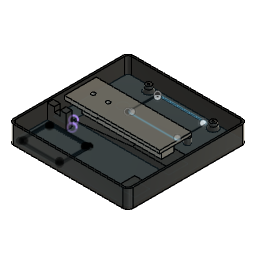
ESPressoScale_Mavin_NA27 (Autodesk Fusion 360 design; units mm, degrees)
Autodesk Fusion 360 part; units mm, degrees
note: some values were not read from the file. Set by a fixed rule: which face or edge a step refers to.
sketch "Skizze1" plane through (0, 0, 0) normal (0, 0, 1) x (1, 0, 0)
  line L0 (-40, 6.35) -> (40, 6.35)
  line L1 (40, 6.35) -> (40, -6.35)
  line L2 (40, -6.35) -> (-40, -6.35)
  line L3 (-40, -6.35) -> (-40, 6.35)
  circle A0 centre (-35, 0.002) radius 2
  circle A1 centre (-20, 0.002) radius 2
  circle A2 centre (35, 0.002) radius 2.5
  circle A3 centre (20, 0.002) radius 2.5
  dimension "d1" = 80
  dimension "d2" = 12.7
  dimension "d3" = 6.35
  dimension "d4" = 40
  dimension "d5" = 4
  dimension "d6" = 5
  dimension "d7" = 4
  dimension "d8" = 20
  dimension "d9" = 5
  dimension "d10" = 5
  dimension "d11" = 5
  dimension "d12" = 20
  constraint horizontal L0
  constraint vertical L1
  constraint horizontal L2
  constraint vertical L3
  measures "d1" distance of L0.start L0.end
  measures "d2" distance of L0.start L2.end
  measures "d3" distance of origin L0
  measures "d4" distance of origin L1
  measures "d5" diameter of A0
  measures "d6" distance of L3 A0.centre
  measures "d7" diameter of A1
  measures "d8" distance of L3 A1.centre
  measures "d9" diameter of A2
  measures "d10" distance of L1 A2.centre
  measures "d11" diameter of A3
  measures "d12" distance of L1 A3.centre
extrude "Extrusion1" add sketch "Skizze1" along normal blind 12.7 makes body 1
copy_body "Körper->Berechn1" bodies 1 removing the originals makes body 2 in component "300gWaegezelle"
sketch "Skizze2" plane through (0, 0, 0) normal (0, 0, 1) x (1, 0, 0)
  line L0 (-65, 65) -> (65, 65)
  line L1 (65, 65) -> (65, -65)
  line L2 (65, -65) -> (-65, -65)
  line L3 (-65, -65) -> (-65, 65)
  dimension "d15" = 130
  dimension "d16" = 130
  dimension "d17" = 65
  dimension "d18" = 65
  constraint horizontal L0
  constraint vertical L1
  constraint horizontal L2
  constraint vertical L3
  measures "d15" distance of L0.start L0.end
  measures "d16" distance of L0.start L2.end
  measures "d17" distance of origin L0
  measures "d18" distance of origin L3
ref_plane "Arbeitsebene1" through (0, 0, 25) normal (0, 0, 1) x (1, 0, 0)
extrude "Extrusion2" add sketch "Skizze2" against normal blind 20 from surface at 25 separate body makes body 3
fillet "Abrundung1" radius 5 8 edges at (-65, 0, 25) (0, 65, 25) (65, 0, 25) (0, -65, 25) (65, -65, 15) (-65, -65, 15) (-65, 65, 15) (65, 65, 15) on bodies 3
shell "Schale1" thickness 3 removed faces 1 at (-23.3333, -21.6667, 5) on bodies 3
extrude "Extrusion3" add 1 faces at (-20, 20, 22) along direction (0, 0, 1) blind 18 from surface at -22 on bodies 3 bodies 3 makes body 4
fillet "Abrundung2" radius 5 4 edges at (60, 60, 9) (-60, 60, 9) (-60, -60, 9) (60, -60, 9) on bodies 4
shell "Schale2" thickness 1.6 outward thickness 0.2 removed faces 1 at (18.3333, -20, 18) on bodies 4
move_body "Verschieben1" bodies 2 to x (1, 0, 0) y (0, 1, 0) z (0, 0, 1) at (0, 0, 8) in component "300gWaegezelle"
sketch "Skizze3" plane through (0, 0, 25) normal (0, 0, 1) x (-1, 0, 0)
  line L0 (60, 60) -> (-60, 60)
  line L1 (-60, 60) -> (-60, -60)
  line L2 (-60, -60) -> (60, -60)
  line L3 (60, -60) -> (60, 60)
  circle A0 centre (0, 0) radius 22
  line L4 (45, 35) -> (31, 35)
  line L5 (31, 35) -> (31, 53)
  line L6 (31, 53) -> (45, 53)
  line L7 (45, 53) -> (45, 35)
  line L8 (-45, 35) -> (-31, 35)
  line L9 (-31, 35) -> (-31, 53)
  line L10 (-31, 53) -> (-45, 53)
  line L11 (-45, 53) -> (-45, 35)
  line L12 (12, 38) -> (-12, 38)
  line L13 (-12, 38) -> (-12, 53)
  line L14 (-12, 53) -> (12, 53)
  line L15 (12, 53) -> (12, 38)
  line L16 (12, 53) -> (-15, 53)
  line L17 (20, 33) -> (-20, 33)
  line L18 (-20, 33) -> (-20, 29)
  line L19 (-20, 29) -> (20, 29)
  line L20 (20, 29) -> (20, 33)
  dimension "d33" = 44
  dimension "d39" = 14
  dimension "d40" = 18
  dimension "d41" = 15
  dimension "d42" = 95
  dimension "d43" = 14
  dimension "d44" = 18
  dimension "d45" = 95
  dimension "d46" = 15
  dimension "d47" = 24
  dimension "d48" = 15
  dimension "d49" = 12
  dimension "d50" = 98
  dimension "d93" = 7
  dimension "d94" = 7
  dimension "d111" = 40
  dimension "d112" = 4
  dimension "d113" = 20
  dimension "d114" = 20
  constraint coincident A0.centre origin
  constraint horizontal L4
  constraint vertical L5
  constraint horizontal L6
  constraint vertical L7
  constraint horizontal L8
  constraint vertical L9
  constraint horizontal L10
  constraint vertical L11
  constraint horizontal L12
  constraint vertical L13
  constraint horizontal L14
  constraint vertical L15
  constraint horizontal L16
  constraint horizontal L17
  constraint vertical L18
  constraint horizontal L19
  constraint vertical L20
  measures "d33" diameter of A0
  measures "d39" distance of L4.start L4.end
  measures "d40" distance of L4.start L6.end
  measures "d41" distance of L3 L7
  measures "d42" distance of L2 L4
  measures "d43" distance of L8.start L8.end
  measures "d44" distance of L8.start L10.end
  measures "d45" distance of L2 L8
  measures "d46" distance of L1 L11
  measures "d47" distance of L12.start L12.end
  measures "d48" distance of L12.start L14.end
  measures "d49" distance of A0.centre L15
  measures "d50" distance of L2 L12
  measures "d93" distance of L0 L14
  measures "d94" distance of L0 L6
  measures "d111" distance of L17.start L17.end
  measures "d112" distance of L17.start L19.end
  measures "d113" distance of A0.centre L18
  measures "d114" distance of L16 L17
extrude "Extrusion5" cut sketch "Skizze3" against normal blind 1 contours A0 bodies 3
extrude "Extrusion6" cut sketch "Skizze3" against normal blind 10 contours L12 L13 L14 L15 L16 bodies 3
extrude "Extrusion7" cut sketch "Skizze3" along normal blind 1.8 from surface at -3 contours L4 L5 L6 L7 | L8 L9 L10 L11 bodies 3
sketch "Skizze4" plane through (0, 0, 1.6) normal (0, 0, 1) x (-1, 0, 0)
  arc A0 (-55, 58.4) -> (-58.4, 55) centre (-55, 55) ccw
  line L0 (-58.4, 55) -> (-58.4, -55)
  arc A1 (-58.4, -55) -> (-55, -58.4) centre (-55, -55) ccw
  line L1 (-55, -58.4) -> (55, -58.4)
  arc A2 (55, -58.4) -> (58.4, -55) centre (55, -55) ccw
  line L2 (58.4, -55) -> (58.4, 55)
  arc A3 (58.4, 55) -> (55, 58.4) centre (55, 55) ccw
  line L3 (55, 58.4) -> (-55, 58.4)
  line L4 (-48.8958, 7.8489) -> (-13.942, 7.8489)
  line L5 (-13.942, 7.8489) -> (-13.942, -7.6745)
  line L6 (-13.942, -7.6745) -> (-48.8958, -7.6745)
  line L7 (-48.8958, -7.6745) -> (-48.8958, 7.8489)
  circle A4 centre (-34.9997, -0.0031) radius 2.75
  circle A5 centre (-19.9963, -0.0044) radius 2.75
  circle A6 centre (-32.5, -53.4) radius 1
  circle A7 centre (-32.5, -53.4) radius 3
  circle A8 centre (32.5, -53.4) radius 1
  circle A9 centre (32.5, -53.4) radius 3
  circle A10 centre (-32.5, -27.4) radius 1
  circle A11 centre (-32.5, -27.4) radius 3
  circle A12 centre (32.5, -27.4) radius 1
  circle A13 centre (32.5, -27.4) radius 3
  line L8 (-53.4, 46.6) -> (-38.4, 46.6)
  line L9 (-38.4, 46.6) -> (-38.4, 31.6)
  line L10 (-38.4, 31.6) -> (-53.4, 31.6)
  line L11 (-53.4, 31.6) -> (-53.4, 46.6)
  line L12 (-55.4, 48.6) -> (-36.4, 48.6)
  line L13 (-36.4, 48.6) -> (-36.4, 29.6)
  line L14 (-36.4, 29.6) -> (-55.4, 29.6)
  line L15 (-55.4, 29.6) -> (-55.4, 48.6)
  line L16 (57.4, 23) -> (37.4, 23)
  line L17 (37.4, 23) -> (37.4, 17)
  line L18 (37.4, 17) -> (57.4, 17)
  line L19 (57.4, 17) -> (57.4, 23)
  line L20 (51.4, 23) -> (45.4, 23)
  line L21 (45.4, 23) -> (45.4, 17)
  line L22 (45.4, 17) -> (51.4, 17)
  line L23 (51.4, 17) -> (51.4, 23)
  circle A14 centre (-34.9997, -0.0031) radius 5.25
  circle A15 centre (-19.9963, -0.0044) radius 5.25
  dimension "d56" = 5.5
  dimension "d57" = 5.5
  dimension "d58" = 2
  dimension "d59" = 32.5
  dimension "d60" = 6
  dimension "d63" = 65
  dimension "d64" = 26
  dimension "d72" = 15
  dimension "d73" = 15
  dimension "d74" = 5
  dimension "d75" = 90
  dimension "d76" = 96.8
  dimension "d77" = -2
  dimension "d80" = 5
  dimension "d81" = 20
  dimension "d82" = 6
  dimension "d83" = 23
  dimension "d84" = 1
  dimension "d85" = 6
  dimension "d86" = 6
  dimension "d118" = 10.5
  dimension "d119" = 10.5
  constraint horizontal L4
  constraint vertical L5
  constraint horizontal L6
  constraint vertical L7
  constraint concentric A6 A7
  constraint horizontal L8
  constraint vertical L9
  constraint horizontal L10
  constraint vertical L11
  constraint horizontal L16
  constraint vertical L17
  constraint horizontal L18
  constraint vertical L19
  constraint horizontal L20
  constraint vertical L21
  constraint horizontal L22
  constraint vertical L23
  constraint coincident L16 L20.start
  constraint concentric A4 A14
  constraint concentric A5 A15
  measures "d56" diameter of A4
  measures "d57" diameter of A5
  measures "d58" diameter of A6
  measures "d59" horizontal distance of origin A6.centre
  measures "d60" diameter of A7
  measures "d72" distance of L8.start L8.end
  measures "d73" distance of L8.start L10.end
  measures "d74" distance of L0 L11
  measures "d75" distance of L1 L10
  measures "d76" distance of L2 L9
  measures "d80" distance of L1 A6.centre
  measures "d81" distance of L16.start L16.end
  measures "d82" distance of L16.start L18.end
  measures "d83" distance of origin L16
  measures "d84" distance of L2 L19
  measures "d85" distance of L20.start L20.end
  measures "d86" distance of L19 L23
  measures "d118" diameter of A14
  measures "d119" diameter of A15
extrude "Extrusion1'" add sketch "Skizze4" along normal up to surface (6.4 mm away) separate body contours L4 L5 L6 L7 | A14 | A15 makes body 5 in component "300gWaegezelle"
combine "Kombinieren1" operation add target body 4 tool bodies 5
move_face "Flächen versetzen1" offset 2 1 faces at (25.5932, 7.6745, 3.7333) on bodies 4
move_face "Flächen versetzen2" offset 2 1 faces at (48.8958, 3.8333, 3.7333) on bodies 4
move_face "Flächen versetzen3" offset 2 1 faces at (38.5779, -7.8489, 3.7333) on bodies 4
extrude "Extrusion8" add sketch "Skizze4" along normal blind 6 contours A7 | A9 | A11 | A13 bodies 4
extrude "Extrusion9" add sketch "Skizze4" along normal blind 4 contours L8 L9 L10 L11 bodies 4
extrude "Extrusion10" add sketch "Skizze4" along normal blind 15 contours L16 L18 L19 L23 | L16 L17 L18 L21 bodies 4
extrude "Extrusion11" add sketch "Skizze4" along normal blind 10 contours L16 L18 L20 L21 L22 L23 bodies 4
sketch "Skizze5" plane through (0, 0, 22) normal (0, 0, -1) x (1, 0, 0)
  line L0 (60, 60) -> (-60, 60)
  line L1 (-60, 60) -> (-60, -60)
  line L2 (-60, -60) -> (60, -60)
  line L3 (60, -60) -> (60, 60)
  line L4 (12, 53) -> (12, 38)
  line L5 (12, 38) -> (-12, 38)
  line L6 (-12, 38) -> (-12, 53)
  line L7 (-45, 53) -> (-31, 53)
  line L8 (-31, 53) -> (-31, 35)
  line L9 (-31, 35) -> (-45, 35)
  line L10 (-45, 35) -> (-45, 53)
  line L11 (45, 53) -> (45, 35)
  line L12 (45, 35) -> (31, 35)
  line L13 (31, 35) -> (31, 53)
  line L14 (31, 53) -> (45, 53)
  line L15 (-17.5, 55) -> (17.5, 55)
  line L16 (17.5, 55) -> (17.5, 35)
  line L17 (17.5, 35) -> (-17.5, 35)
  line L18 (-17.5, 35) -> (-17.5, 55)
  line L19 (-12, 53) -> (12, 53)
  line L20 (-17.5, 55) -> (17.5, 55)
  line L21 (17.5, 55) -> (17.5, 63)
  line L22 (17.5, 63) -> (-17.5, 63)
  line L23 (-17.5, 63) -> (-17.5, 55)
  dimension "d102" = 35
  dimension "d103" = 20
  dimension "d104" = 17.5
  dimension "d105" = 5
  dimension "d125" = 8
  constraint horizontal L15
  constraint vertical L16
  constraint horizontal L17
  constraint vertical L18
  constraint horizontal L20
  constraint vertical L21
  constraint horizontal L22
  constraint vertical L23
  measures "d102" distance of L15.start L15.end
  measures "d103" distance of L15.start L17.end
  measures "d104" distance of origin L16
  measures "d105" distance of L0 L15
  measures "d125" distance of L15.start L22.end
extrude "Extrusion13" cut sketch "Skizze5" against normal blind 1.5 contours L15 L16 L17 L18 L20 bodies 3
extrude "Extrusion14" add sketch "Skizze3" against normal blind 1.5 from surface at -3 contours L17 L18 L19 L20 bodies 3
chamfer "Fase1" distance 59 distance2 6.4 1 edges at (13.942, -0.0872, 1.6) measured on face at (-18, -42.6667, 1.6) on bodies 4
extrude "Extrusion15" cut sketch "Skizze4" along normal blind 5 from surface at -1.8 contours A4 | A5 | A14 | A15 bodies 4
extrude "Extrusion16" add sketch "Skizze5" along normal blind 1.5 contours L0 L15 L20 L21 L23 | L0 L21 L22 L23 bodies 3
extrude "Extrusion17" add sketch "Skizze5" against normal blind 0.7 separate body contours L15 L16 L17 L18 L20 makes body 6
extrude "Extrusion18" add sketch "Skizze5" against normal blind 2 contours L4 L5 L6 L19 bodies 6
extrude "Extrusion19" cut 1 faces at (-37.4, -21, 11.6) along direction (-1, 0, 0) blind 2 on bodies 4 bodies 4
chamfer "Fase3" distance 2 distance2 3 3 edges at (-29.703, 52.3152, 1.6) (-29.703, 26.3152, 1.6) (35.297, 52.3152, 1.6) measured on face at (-18.6667, -42.6667, 1.6) measured on face at (-18.6667, -42.6667, 1.6) measured on face at (-18.6667, -42.6667, 1.6) on bodies 4
extrude "Extrusion20" add 1 faces at (-57.4, -19, 11.6) along direction (-1, 0, 0) up to surface (1 mm away) on bodies 4 bodies 4
sketch "Skizze7" plane through (0, 0, 1.6) normal (0, 0, 1) x (-1, 0, 0)
  line L0 (45.058, -9.6745) -> (-50.8958, -9.6745)
  line L1 (-50.8958, -9.6745) -> (-50.8958, 9.8489)
  line L2 (-50.8958, 9.8489) -> (45.058, 9.8489)
  line L3 (45.058, 9.8489) -> (45.058, -9.6745)
  line L4 (-53.4, 31.6) -> (-53.4, 46.6)
  line L5 (-53.4, 46.6) -> (-38.4, 46.6)
  line L6 (-38.4, 46.6) -> (-38.4, 31.6)
  line L7 (-38.4, 31.6) -> (-53.4, 31.6)
  line L8 (39.4, 23) -> (58.4, 23)
  line L9 (58.4, 23) -> (58.4, 55)
  arc A0 (58.4, 55) -> (55, 58.4) centre (55, 55) ccw
  line L10 (55, 58.4) -> (-55, 58.4)
  arc A1 (-55, 58.4) -> (-58.4, 55) centre (-55, 55) ccw
  line L11 (-58.4, 55) -> (-58.4, -55)
  arc A2 (-58.4, -55) -> (-55, -58.4) centre (-55, -55) ccw
  line L12 (-55, -58.4) -> (-32.5, -58.4)
  circle A3 centre (-32.5, -53.4) radius 5
  line L13 (-32.5, -58.4) -> (32.5, -58.4)
  circle A4 centre (32.5, -53.4) radius 5
  line L14 (32.5, -58.4) -> (55, -58.4)
  arc A5 (55, -58.4) -> (58.4, -55) centre (55, -55) ccw
  line L15 (58.4, -55) -> (58.4, 17)
  line L16 (58.4, 17) -> (39.4, 17)
  line L17 (39.4, 17) -> (39.4, 23)
  circle A6 centre (-32.5, -27.4) radius 3
  circle A7 centre (32.5, -27.4) radius 5
  line L18 (23, -54.7754) -> (-23, -54.7754)
  line L19 (-25, -52.7754) -> (-25, -26.7754)
  line L20 (-23, -24.7754) -> (23, -24.7754)
  line L21 (25, -26.7754) -> (25, -52.7754)
  line L22 (16, 55) -> (52, 55)
  line L23 (54, 53) -> (54, 27)
  line L24 (52, 25) -> (16, 25)
  line L25 (14, 27) -> (14, 53)
  arc A8 (52, 25) -> (54, 27) centre (52, 27) ccw
  arc A9 (14, 27) -> (16, 25) centre (16, 27) ccw
  arc A10 (16, 55) -> (14, 53) centre (16, 53) ccw
  arc A11 (54, 53) -> (52, 55) centre (52, 53) ccw
  line L26 (52, 26) -> (16, 26)
  arc A12 (15, 27) -> (16, 26) centre (16, 27) ccw
  line L27 (15, 27) -> (15, 53)
  arc A13 (16, 54) -> (15, 53) centre (16, 53) ccw
  line L28 (16, 54) -> (52, 54)
  arc A14 (53, 53) -> (52, 54) centre (52, 53) ccw
  line L29 (53, 53) -> (53, 27)
  arc A15 (52, 26) -> (53, 27) centre (52, 27) ccw
  arc A16 (12.5, 27) -> (16, 23.5) centre (16, 27) ccw
  line L30 (52, 23.5) -> (16, 23.5)
  arc A17 (52, 23.5) -> (55.5, 27) centre (52, 27) ccw
  line L31 (55.5, 53) -> (55.5, 27)
  arc A18 (55.5, 53) -> (52, 56.5) centre (52, 53) ccw
  line L32 (16, 56.5) -> (52, 56.5)
  arc A19 (16, 56.5) -> (12.5, 53) centre (16, 53) ccw
  line L33 (12.5, 27) -> (12.5, 53)
  arc A20 (23, -54.7754) -> (25, -52.7754) centre (23, -52.7754) ccw
  arc A21 (-25, -52.7754) -> (-23, -54.7754) centre (-23, -52.7754) ccw
  arc A22 (-23, -24.7754) -> (-25, -26.7754) centre (-23, -26.7754) ccw
  arc A23 (25, -26.7754) -> (23, -24.7754) centre (23, -26.7754) ccw
  point P0 (25, -54.7754)
  point P1 (25, -24.7754)
  point P2 (14, 55)
  point P3 (54, 55)
  point P4 (14, 25)
  dimension "d140" = 30
  dimension "d141" = 50
  dimension "d142" = 25
  dimension "d143" = 40
  dimension "d144" = 30
  dimension "d146" = 1
  dimension "d152" = 2
  dimension "d153" = 25
  dimension "d154" = 4.4
  dimension "d155" = 72.4
  dimension "d156" = -1.5
  dimension "d157" = 2
  dimension "d179" = 14
  constraint horizontal L18
  constraint vertical L19
  constraint horizontal L20
  constraint vertical L21
  constraint horizontal L22
  constraint vertical L23
  constraint horizontal L24
  constraint vertical L25
  constraint tangent L23 A8
  constraint tangent L24 A8
  constraint coincident P4 L24
  constraint coincident P4 L25
  constraint tangent L24 A9
  constraint tangent L25 A9
  constraint equal A8 A9
  constraint coincident P2 L22
  constraint coincident P2 L25
  constraint tangent L22 A10
  constraint tangent L25 A10
  constraint equal A8 A10
  constraint coincident P3 L22
  constraint coincident P3 L23
  constraint tangent L22 A11
  constraint tangent L23 A11
  constraint equal A8 A11
  constraint coincident P0 L18
  constraint coincident P0 L21
  constraint tangent L18 A20
  constraint tangent L21 A20
  constraint tangent L18 A21
  constraint tangent L19 A21
  constraint equal A20 A21
  constraint tangent L19 A22
  constraint tangent L20 A22
  constraint equal A20 A22
  constraint coincident P1 L20
  constraint coincident P1 L21
  constraint tangent L20 A23
  constraint tangent L21 A23
  constraint equal A20 A23
  measures "d140" distance of P0 P1
  measures "d141" distance of L19 L21
  measures "d142" horizontal distance of origin P0
  measures "d143" distance of P2 P3
  measures "d144" distance of P2 P4
  measures "d152" radius of A8
  measures "d153" distance of origin L24
  measures "d154" distance of L10 L28
  measures "d155" distance of L11 L25
  measures "d157" radius of A20
  measures "d179" distance of origin L25
extrude "Extrusion24" cut 1 faces at (-5.8152, 3.0625, 24) along direction (0, 0, -1) blind 0.5 on bodies 3 bodies 3
extrude "Extrusion21" cut sketch "Skizze7" against normal blind 1 contours L18 L19 L20 L21 A20 A21 A22 A23 bodies 4
extrude "Extrusion22" cut sketch "Skizze7" along normal blind 0.2 from surface at -1.8 contours L22 L23 L24 L25 A8 A9 A10 A11 bodies 4
extrude "Extrusion23" cut sketch "Skizze7" against normal blind 0.8 contours L18 L19 L20 L21 A20 A21 A22 A23 | L22 L23 L24 L25 A8 A9 A10 A11 | L26 A12 L27 A13 L28 A14 L29 A15 | A16 L30 A17 L31 A18 L32 A19 L33 bodies 4
extrude "Extrusion25" add 1 faces at (50.8958, 3.1667, 3.7333) along direction (1, 0, 0) up to surface (7.5042 mm away) on bodies 4 bodies 4
sketch "Skizze8" plane through (0, 0, 20.7) normal (0, 0, 1) x (-1, 0, 0)
  circle A0 centre (-35, -0.002) radius 2.5
  circle A1 centre (35, -0.002) radius 2
  circle A2 centre (20, -0.002) radius 2
  circle A3 centre (-20, -0.002) radius 2.5
  line L0 (40, 6.35) -> (-40, 6.35)
  line L1 (-40, 6.35) -> (-40, -6.35)
  line L2 (-40, -6.35) -> (40, -6.35)
  line L3 (40, -6.35) -> (40, 6.35)
  line L4 (48, 16) -> (-48, 16)
  line L5 (-48, 16) -> (-48, -16)
  line L6 (-48, -16) -> (48, -16)
  line L7 (48, -16) -> (48, 16)
  circle A4 centre (20, -0.002) radius 2
  circle A5 centre (35, -0.002) radius 2
  line L8 (48, 16) -> (15, 16)
  line L9 (15, 16) -> (15, -16)
  line L10 (15, -16) -> (48, -16)
  line L11 (48, -16) -> (48, 16)
  dimension "d163" = 32
  dimension "d164" = 96
  dimension "d165" = 16
  dimension "d166" = 48
  dimension "d169" = 33
  dimension "d177" = 13
  dimension "d178" = 28
  constraint horizontal L4
  constraint vertical L5
  constraint horizontal L6
  constraint vertical L7
  constraint concentric A2 A4
  constraint concentric A1 A5
  constraint horizontal L8
  constraint vertical L9
  constraint horizontal L10
  constraint vertical L11
  measures "d163" distance of L4 L6
  measures "d164" distance of L5 L7
  measures "d165" distance of origin L4
  measures "d166" distance of origin L7
  measures "d169" distance of L4.start L8.end
  measures "d177" distance of L7 A1.centre
  measures "d178" distance of L7 A2.centre
extrude "Extrusion26" add sketch "Skizze8" along normal blind 3 from surface at 1 separate body contours A0 | A3 | L0 L2 L3 L9 | L0 L2 L3 L4 L6 L7 L8 L9 L10 L11 | L0 L1 L2 L9 | L0 L1 L2 L4 L5 L6 L9 makes body 7
extrude "Extrusion27" add sketch "Skizze8" along normal up to surface (1 mm away) contours L0 L2 L3 L9 | L0 L2 L3 L4 L6 L7 L8 L9 L10 L11 bodies 7
move_body "Verschieben1'" bodies 3 to x (1, 0, 0) y (0, 1, 0) z (0, 0, 1) at (0, 0, 2.7)
component "300gWaegezelle" placed x (1, 0, 0) y (0, 1, 0) z (0, 0, 1) at (0, 0, 0)
hidden bodies 3 6
equation "d3 = ( 12.7 / 2 ) * 1 mm"
equation "d4 = ( 80 / 2 ) * 1 mm"
equation "d17 = ( 130 / 2 ) * 1 mm"
equation "d18 = ( 130 / 2 ) * 1 mm"
equation "d49 = ( 24 / 2 ) * 1 mm"
equation "d59 = ( 65 / 2 ) * 1 mm"
equation "d89 = 15 mm - 5 mm"
equation "d104 = ( 35 / 2 ) * 1 mm"
equation "d165 = ( 32 / 2 ) * 1 mm"
equation "d166 = ( 96 / 2 ) * 1 mm"
named bodies: "300gWaegezelle", "Top", "Bottom", "Glas", "Carrier"
